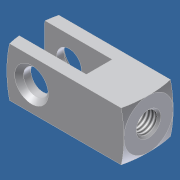
# Autodesk Inventor part: D-14055
Saved by Autodesk Inventor 2012 (Build 160160000, 160)
## iProperties
Category: PARTsolutions
Created: 2013-01-19
Part Number: D-14055
Catalog Web Link: www.cadenas.de
Description: Piston Rod Clevis for Original Line Cylinders - Body -
Document SubType Name: Modeling
Designer: PARTsolutions
Material: Default
Density: 1 g/cm^3
Mass: 2.86229 g
Surface Area: 21.8011 cm^2
Volume: 2.86229 cm^3
NB: D-14055
NN: Piston Rod Clevis for Original Line Cylinders - Body
NBSYN: $PN.
LINA: D-14055
PN: D-14055
L: 1.18800000
L1: 0.93800000
L2: 0.50000000
W: 0.26250000
W1: 0.50000000
DIA1: 0.25150000
DIA1CS: 0.04500000
DIA2: 0.50000000
DIA3: 0.21300000
CS: 90.00000000
CDP: 0.03000000
AN: 30.00000000
NDM: 0.25000000
CODE: UNF
NDMDP: 0.44000000
COLOR: 0.75,0.75,0.75,0.00
KT: DUMMY
SUPPLIER: Bimba
ARTICLENO: D-14055
BOMINFO: D-14055
CREATOR: CADENAS GmbH
PSOL_IDENT_0: {\\10.0.0.242\data_v9\23d-libs\bimba\bimba\bimba_imperial\bimba_full_line\original_line_cylinders\ac
PSOL_IDENT_1: cessories\piston_rod_clevis_body.prj},202 {VTYP=3D},{NB=D-14055},{LINA=D-14055},{NN=Piston Rod Clevi
PSOL_IDENT_2: s for Original Line Cylinders - Body},{DATE=06.12.2012 09:37:17},{GEOMDATE=06.12.2012 07:16:06},{VER
PSOL_IDENT_3: SION=},{LINEID=30},{LINESUBID=-1},{WBVAR=}  {NB=D-14055},{LINA=D-14055},{KT=DUMMY},{PN=D-14055},{L=1
PSOL_IDENT_4: .18800000},{L1=0.93800000},{L2=0.50000000},{W=0.26250000},{W1=0.50000000},{DIA1=0.25150000},{DIA1CS=
PSOL_IDENT_5: 0.04500000},{DIA2=0.50000000},{DIA3=0.21300000},{CS=90.00000000},{CDP=0.03000000},{AN=30.00000000},{
PSOL_IDENT_6: NDM=0.25000000},{CODE=UNF},{NDMDP=0.44000000},{COLOR=0.75,0.75,0.75,0.00}
Title: D-14055
Author: Cadenas PARTsolutions
Autodesk Inventor part; units mm, degrees
sketch "Sketch_1" plane through (0, 0, 0) normal (0, 0, 1) x (1, 0, 0)
  line L0 (-6.35, 6.35) -> (-6.35, -6.35)
  line L1 (-6.35, -6.35) -> (23.8252, -6.35)
  line L2 (23.8252, -6.35) -> (23.8252, 6.35)
  line L3 (23.8252, 6.35) -> (-6.35, 6.35)
  constraints: 8 end point
extrude "Extrusion1" add sketch "Sketch_1" along normal mid plane 12.7
sketch "Sketch_2" plane through (0, 0, 0) normal (0, 1, 0) x (-1, 0, 0)
  line L0 (6.35, -3.3338) -> (6.35, 3.3338)
  line L1 (6.35, 3.3338) -> (-11.1252, 3.3338)
  line L2 (-11.1252, 3.3338) -> (-11.1252, -3.3338)
  line L3 (-11.1252, -3.3338) -> (6.35, -3.3338)
  constraints: 8 end point
extrude "Extrusion2" cut sketch "Sketch_2" along normal mid plane 12.7
sketch "Sketch_3" plane through (0, 0, 0) normal (0, 0, 1) x (1, 0, 0)
  line L0 (23.8252, 0) -> (12.6492, 0)
  line L1 (12.6492, 0) -> (12.6492, 2.6835)
  line L2 (12.6492, 2.6835) -> (23.3337, 2.6835)
  line L3 (23.3337, 2.6835) -> (23.8252, 3.175)
  line L4 (23.8252, 3.175) -> (23.8252, 0)
  line L5 (23.8252, 0) -> (12.6492, 0)
  constraints: 12 end point
revolve "Revolution1" cut sketch "Sketch_3" angle 360 about axis through (23.8252, 0, 0) along (1, 0, 0)
thread "Thread1" size "1/4-27 UNS" class "2B" standard "ANSI Unified Screw Threads" full length
sketch "Sketch_4" plane through (0, 0, 0) normal (0, 0, 1) x (1, 0, 0)
  line L0 (12.6492, 0) -> (11.1252, 0)
  line L1 (11.1252, 0) -> (11.1252, 2.7051)
  line L2 (11.1252, 2.7051) -> (12.6492, 2.7051)
  line L3 (12.6492, 2.7051) -> (12.6492, 0)
  line L4 (12.6492, 0) -> (11.1252, 0)
  constraints: 10 end point
revolve "Revolution2" cut sketch "Sketch_4" angle 360 about axis through (12.6492, 0, 0) along (1, 0, 0)
sketch "Sketch_5" plane through (0, 0, 0) normal (1, 0, 0) x (0, 1, 0)
  line L0 (0, -6.35) -> (0, 6.35)
  line L1 (0, 6.35) -> (4.337, 6.35)
  line L2 (4.337, 6.35) -> (3.194, 5.207)
  line L3 (3.194, 5.207) -> (3.194, -5.207)
  line L4 (3.194, -5.207) -> (4.337, -6.35)
  line L5 (4.337, -6.35) -> (0, -6.35)
  line L6 (0, -6.35) -> (0, 6.35)
  constraints: 14 end point
revolve "Revolution3" cut sketch "Sketch_5" angle 360 about axis through (0, 0, -6.35) along (0, 0, -1)
sketch "Sketch_9" plane through (0, 0, 0) normal (0, 0, 1) x (1, 0, 0)
  line L0 (30.1752, 0) -> (23.8252, 0)
  line L1 (23.8252, 0) -> (23.8252, 6.35)
  arc A0 (23.8252, 6.35) -> (21.2852, 12.7) centre (6.6802, 3.175) ccw
  line L2 (21.2852, 12.7) -> (30.1752, 12.7)
  line L3 (30.1752, 12.7) -> (30.1752, 0)
  line L4 (30.1752, 0) -> (23.8252, 0)
  constraints: 10 end point, 2 point on circle, 1 centre point
revolve "Revolution4" cut sketch "Sketch_9" angle 360 about axis through (30.1752, 0, 0) along (1, 0, 0)
sketch "Sketch_10" plane through (0, 0, 0) normal (0, 0, 1) x (1, 0, 0)
  line L0 (-6.35, 0) -> (-12.7, 0)
  line L1 (-12.7, 0) -> (-12.7, 12.7)
  line L2 (-12.7, 12.7) -> (-3.81, 12.7)
  arc A0 (-3.81, 12.7) -> (-6.35, 6.35) centre (10.795, 3.175) ccw
  line L3 (-6.35, 6.35) -> (-6.35, 0)
  line L4 (-6.35, 0) -> (-12.7, 0)
  constraints: 10 end point, 2 point on circle, 1 centre point
revolve "Revolution5" cut sketch "Sketch_10" angle 360 about axis through (-6.35, 0, 0) along (1, 0, 0)
ref_plane "th1_XY" through (23.8252, 3.175, 0) normal (0, 0, 1) x (1, 0, 0)
ref_plane "th1_YZ" through (23.8252, 3.175, 0) normal (1, 0, 0) x (0, 1, 0)
ref_plane "th1_ZX" through (23.8252, 3.175, 0) normal (0, 1, 0) x (0, 0, 1)
ref_plane "th2_XY" through (23.8252, -3.175, 0) normal (0, 0, 1) x (1, 0, 0)
ref_plane "th2_YZ" through (23.8252, -3.175, 0) normal (1, 0, 0) x (0, 1, 0)
ref_plane "th2_ZX" through (23.8252, -3.175, 0) normal (0, 1, 0) x (0, 0, 1)
ref_plane "rod_clevis_body_XY" through (0, 0, 0) normal (0, 0, 1) x (1, 0, 0)
ref_plane "rod_clevis_body_YZ" through (0, 0, 0) normal (1, 0, 0) x (0, 1, 0)
ref_plane "rod_clevis_body_ZX" through (0, 0, 0) normal (0, 1, 0) x (0, 0, 1)
ref_plane "piston_rod_clevis_XY" through (23.8252, 0, 0) normal (1, 0, 0) x (0, 0, -1)
ref_plane "piston_rod_clevis_YZ" through (23.8252, 0, 0) normal (0, 0, -1) x (0, 1, 0)
ref_plane "piston_rod_clevis_ZX" through (23.8252, 0, 0) normal (0, 1, 0) x (1, 0, 0)
ref_plane "dummy_XY" through (0, 0, 0) normal (0, 0, 1) x (1, 0, 0)
ref_plane "dummy_YZ" through (0, 0, 0) normal (1, 0, 0) x (0, 1, 0)
ref_plane "dummy_ZX" through (0, 0, 0) normal (0, 1, 0) x (0, 0, 1)
ref_plane "l11_XY" through (23.8252, 6.35, 0) normal (0, 0, 1) x (1, 0, 0)
ref_plane "l11_YZ" through (23.8252, 6.35, 0) normal (1, 0, 0) x (0, 1, 0)
ref_plane "l11_ZX" through (23.8252, 6.35, 0) normal (0, 1, 0) x (0, 0, 1)
ref_plane "l12_XY" through (0, 6.35, 0) normal (0, 0, 1) x (1, 0, 0)
ref_plane "l12_YZ" through (0, 6.35, 0) normal (1, 0, 0) x (0, 1, 0)
ref_plane "l12_ZX" through (0, 6.35, 0) normal (0, 1, 0) x (0, 0, 1)
ref_plane "l1_XY" through (23.8252, 6.35, 0) normal (0, 0, 1) x (1, 0, 0)
ref_plane "l1_YZ" through (23.8252, 6.35, 0) normal (1, 0, 0) x (0, 1, 0)
ref_plane "l1_ZX" through (23.8252, 6.35, 0) normal (0, 1, 0) x (0, 0, 1)
ref_plane "h1_XY" through (-6.35, 6.35, 0) normal (0, 0, 1) x (1, 0, 0)
ref_plane "h1_YZ" through (-6.35, 6.35, 0) normal (1, 0, 0) x (0, 1, 0)
ref_plane "h1_ZX" through (-6.35, 6.35, 0) normal (0, 1, 0) x (0, 0, 1)
ref_plane "l2_XY" through (-6.35, 6.35, 0) normal (0, 0, 1) x (1, 0, 0)
ref_plane "l2_YZ" through (-6.35, 6.35, 0) normal (1, 0, 0) x (0, 1, 0)
ref_plane "l2_ZX" through (-6.35, 6.35, 0) normal (0, 1, 0) x (0, 0, 1)
ref_plane "h2_XY" through (-6.35, -6.35, 0) normal (0, 0, 1) x (1, 0, 0)
ref_plane "h2_YZ" through (-6.35, -6.35, 0) normal (1, 0, 0) x (0, 1, 0)
ref_plane "h2_ZX" through (-6.35, -6.35, 0) normal (0, 1, 0) x (0, 0, 1)
ref_plane "w11_XY" through (-6.35, 0, -3.3338) normal (0, 1, 0) x (1, 0, 0)
ref_plane "w11_YZ" through (-6.35, 0, -3.3338) normal (1, 0, 0) x (0, 0, -1)
ref_plane "w11_ZX" through (-6.35, 0, -3.3338) normal (0, 0, -1) x (0, 1, 0)
ref_plane "w12_XY" through (-6.35, 0, 3.3338) normal (0, 1, 0) x (1, 0, 0)
ref_plane "w12_YZ" through (-6.35, 0, 3.3338) normal (1, 0, 0) x (0, 0, -1)
ref_plane "w12_ZX" through (-6.35, 0, 3.3338) normal (0, 0, -1) x (0, 1, 0)
ref_plane "l21_XY" through (23.8252, 0, 0) normal (0, 1, 0) x (1, 0, 0)
ref_plane "l21_YZ" through (23.8252, 0, 0) normal (1, 0, 0) x (0, 0, -1)
ref_plane "l21_ZX" through (23.8252, 0, 0) normal (0, 0, -1) x (0, 1, 0)
ref_plane "l22_XY" through (11.1252, 0, 0) normal (0, 1, 0) x (1, 0, 0)
ref_plane "l22_YZ" through (11.1252, 0, 0) normal (1, 0, 0) x (0, 0, -1)
ref_plane "l22_ZX" through (11.1252, 0, 0) normal (0, 0, -1) x (0, 1, 0)
ref_plane "w1_XY" through (23.8252, 0, -6.35) normal (0, 1, 0) x (1, 0, 0)
ref_plane "w1_YZ" through (23.8252, 0, -6.35) normal (1, 0, 0) x (0, 0, -1)
ref_plane "w1_ZX" through (23.8252, 0, -6.35) normal (0, 0, -1) x (0, 1, 0)
ref_plane "w2_XY" through (23.8252, 0, 6.35) normal (0, 1, 0) x (1, 0, 0)
ref_plane "w2_YZ" through (23.8252, 0, 6.35) normal (1, 0, 0) x (0, 0, -1)
ref_plane "w2_ZX" through (23.8252, 0, 6.35) normal (0, 0, -1) x (0, 1, 0)
ref_plane "to_cylinder_XY" through (11.1252, 0, 0) normal (1, 0, 0) x (0, 0, -1)
ref_plane "to_cylinder_YZ" through (11.1252, 0, 0) normal (0, 0, -1) x (0, 1, 0)
ref_plane "to_cylinder_ZX" through (11.1252, 0, 0) normal (0, 1, 0) x (1, 0, 0)
body "Solid1"
